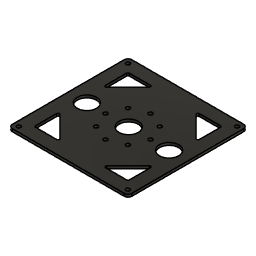
motor-holder (Autodesk Fusion 360 design; units mm, degrees)
Autodesk Fusion 360 part; units mm, degrees
sketch "Sketch1" plane through (0, 0, 0) normal (0, 0, 1) x (1, 0, 0)
  line L0 (-27, 30) -> (60, 30)
  line L1 (63, 27) -> (63, -60)
  line L2 (60, -63) -> (-27, -63)
  line L3 (-30, -60) -> (-30, 27)
  arc A0 (-27, 30) -> (-30, 27) centre (-27, 27) ccw
  arc A1 (63, 27) -> (60, 30) centre (60, 27) ccw
  arc A2 (-30, -60) -> (-27, -63) centre (-27, -60) ccw
  arc A3 (60, -63) -> (63, -60) centre (60, -60) ccw
  point P0 (-30, 30)
  point P1 (63, 30)
  point P2 (-30, -63)
  dimension "d1" = 93
  dimension "d2" = 93
  dimension "d3" = 3
  dimension "d4" = 3
  constraint horizontal L0
  constraint vertical L1
  constraint horizontal L2
  constraint vertical L3
  constraint coincident P0 L0
  constraint coincident P0 L3
  constraint tangent L0 A0
  constraint tangent L3 A0
  constraint coincident P1 L0
  constraint coincident P1 L1
  constraint tangent L0 A1
  constraint tangent L1 A1
  constraint coincident P2 L2
  constraint coincident P2 L3
  constraint tangent L2 A2
  constraint tangent L3 A2
  constraint equal A1 A2
  constraint tangent L1 A3
  constraint tangent L2 A3
  constraint equal A1 A3
  measures "d1" distance of P0 P1
  measures "d2" distance of P0 P2
  measures "d3" radius of A0
  measures "d4" radius of A1
extrude "Extrude1" add sketch "Sketch1" along normal blind 2
sketch "Sketch2" plane through (0, 0, 2) normal (0, 0, 1) x (-1, 0, 0)
  arc A0 (30, 60) -> (27, 63) centre (27, 60) ccw
  line L0 (27, 63) -> (-60, 63)
  arc A1 (-60, 63) -> (-63, 60) centre (-60, 60) ccw
  line L1 (-63, 60) -> (-63, -27)
  arc A2 (-63, -27) -> (-60, -30) centre (-60, -27) ccw
  line L2 (-60, -30) -> (27, -30)
  arc A3 (27, -30) -> (30, -27) centre (27, -27) ccw
  line L3 (30, -27) -> (30, 60)
  point P0 (26, -26)
  point P1 (-59, -26)
  point P2 (26, 59)
  point P3 (-60, 60)
  point P4 (-59, 59)
  point P5 (-57.2336, -24.9323)
  dimension "d18" = 85
  dimension "d19" = 4
  dimension "d20" = 4
  dimension "d21" = 4
  dimension "d22" = 4
  dimension "d23" = 4
  dimension "d24" = 4
  dimension "d25" = 85
  dimension "d26" = 4
  constraint coincident P3 A1.centre
  measures "d18" distance of P0 P1
  measures "d19" distance of L1 P1
  measures "d20" distance of L3 P0
  measures "d21" distance of L2 P0
  measures "d22" distance of L2 P1
  measures "d23" distance of L3 P2
  measures "d24" distance of L0 P2
  measures "d25" horizontal distance of P2 P4
  measures "d26" distance of L0 P4
hole "Hole2" at (59, -59, 2) at (-26, -59, 2) at (-26, 26, 2) at (59, 26, 2) direction (0, 0, -1) diameter 3 depth 2 tip angle 118
sketch "Sketch3" plane through (0, 0, 2) normal (0, 0, 1) x (-1, 0, 0)
  line L0 (-60, -30) -> (27, -30)
  line L1 (30, -27) -> (30, 60)
  line L2 (27, 63) -> (-60, 63)
  point P0 (-16.5, 16.5)
  point P1 (-16.5, -1)
  point P2 (1, 16.5)
  point P3 (-16.5, 34)
  point P4 (-34, 16.5)
  point P5 (-28.8744, 28.8744)
  point P6 (-4.1256, 28.8744)
  point P7 (-4.1256, 4.1256)
  point P8 (-28.8744, 4.1256)
  point P9 (-34, 16.5)
  point P10 (-16.5, 34)
  point P11 (1, 16.5)
  point P12 (-16.5, -1)
  point P13 (-28.8744, 4.1256)
  point P14 (-28.8744, 28.8744)
  point P15 (-4.1256, 28.8744)
  point P16 (-4.1256, 4.1256)
  point P17 (-16.5, -1)
  point P18 (-34, 16.5)
  point P19 (-16.5, 34)
  point P20 (1, 16.5)
  point P21 (-4.1256, 4.1256)
  point P22 (-28.8744, 4.1256)
  point P23 (-28.8744, 28.8744)
  point P24 (-4.1256, 28.8744)
  point P25 (1, 16.5)
  point P26 (-16.5, -1)
  point P27 (-34, 16.5)
  point P28 (-16.5, 34)
  point P29 (-4.1256, 28.8744)
  point P30 (-4.1256, 4.1256)
  point P31 (-28.8744, 4.1256)
  point P32 (-28.8744, 28.8744)
  dimension "d30" = 46.5
  dimension "d31" = 46.5
  dimension "d32" = 17.5
  dimension "d34" = 46.5
  dimension "d35" = 46.5
  dimension "d36" = 46.5
  dimension "d38" = 46.5
  dimension "d39" = 17.5
  dimension "d40" = 17.5
  dimension "d41" = 17.5
  dimension "d47" = 360
  measures "d30" distance of P0 L0
  measures "d31" distance of P0 L1
  measures "d32" horizontal distance of P0 P25
  measures "d34" distance of P26 L1
  measures "d35" distance of P27 L0
  measures "d36" distance of P25 L2
  measures "d38" distance of P28 L1
  measures "d39" distance of P0 P27
  measures "d40" distance of P0 P26
  measures "d41" distance of P0 P28
hole "Hole3" at (16.5, -34, 2) at (-1, -16.5, 2) at (16.5, 1, 2) at (34, -16.5, 2) at (16.5, -34, 2) at (4.1256, -28.8744, 2) at (4.1256, -4.1256, 2) at (28.8744, -28.8744, 2) at (28.8744, -4.1256, 2) direction (0, 0, -1) diameter 3 depth 25 tip angle 118
sketch "Sketch4" plane through (0, 0, 2) normal (0, 0, 1) x (-1, 0, 0)
sketch "Sketch5" plane through (0, 0, 2) normal (0, 0, 1) x (-1, 0, 0)
  circle A0 centre (-28.8744, 28.8744) radius 1.5
  circle A1 centre (-4.1256, 28.8744) radius 1.5
  circle A2 centre (-34, 16.5) radius 1.5
  circle A3 centre (1, 16.5) radius 1.5
  circle A4 centre (-16.5, 34) radius 1.5
  circle A5 centre (-16.5, -1) radius 1.5
  circle A6 centre (-4.1256, 4.1256) radius 1.5
  circle A7 centre (-28.8744, 4.1256) radius 1.5
  circle A8 centre (26, -26) radius 1.5
  circle A9 centre (-59, 59) radius 1.5
  circle A10 centre (26, 59) radius 1.5
  circle A11 centre (-59, -26) radius 1.5
  arc A12 (30, 60) -> (27, 63) centre (27, 60) ccw
  line L0 (27, 63) -> (-60, 63)
  arc A13 (-60, 63) -> (-63, 60) centre (-60, 60) ccw
  line L1 (-63, 60) -> (-63, -27)
  arc A14 (-63, -27) -> (-60, -30) centre (-60, -27) ccw
  line L2 (-60, -30) -> (27, -30)
  arc A15 (27, -30) -> (30, -27) centre (27, -27) ccw
  line L3 (30, -27) -> (30, 60)
  circle A16 centre (15.5, 16.5) radius 7.5
  circle A17 centre (-48.5, 16.5) radius 7.5
  dimension "d48" = 15
  dimension "d49" = 14.5
  dimension "d50" = 46.5
  dimension "d51" = 15
  dimension "d52" = 46.5
  dimension "d53" = 14.5
  measures "d48" diameter of A16
  measures "d49" distance of L3 A16.centre
  measures "d50" distance of L2 A16.centre
  measures "d51" diameter of A17
  measures "d52" distance of L2 A17.centre
  measures "d53" distance of L1 A17.centre
extrude "Extrude2" cut sketch "Sketch5" against normal blind 9 contours A16 | A17
sketch "Sketch6" plane through (0, 0, 2) normal (0, 0, 1) x (-1, 0, 0)
  circle A0 centre (-48.5, 16.5) radius 7.5
  circle A1 centre (15.5, 16.5) radius 7.5
  circle A2 centre (-28.8744, 28.8744) radius 1.5
  circle A3 centre (-4.1256, 28.8744) radius 1.5
  circle A4 centre (-34, 16.5) radius 1.5
  circle A5 centre (1, 16.5) radius 1.5
  circle A6 centre (-16.5, 34) radius 1.5
  circle A7 centre (-16.5, -1) radius 1.5
  circle A8 centre (-4.1256, 4.1256) radius 1.5
  circle A9 centre (-28.8744, 4.1256) radius 1.5
  circle A10 centre (26, -26) radius 1.5
  circle A11 centre (-59, 59) radius 1.5
  circle A12 centre (26, 59) radius 1.5
  circle A13 centre (-59, -26) radius 1.5
  arc A14 (30, 60) -> (27, 63) centre (27, 60) ccw
  line L0 (27, 63) -> (-60, 63)
  arc A15 (-60, 63) -> (-63, 60) centre (-60, 60) ccw
  line L1 (-63, 60) -> (-63, -27)
  arc A16 (-63, -27) -> (-60, -30) centre (-60, -27) ccw
  line L2 (-60, -30) -> (27, -30)
  arc A17 (27, -30) -> (30, -27) centre (27, -27) ccw
  line L3 (30, -27) -> (30, 60)
sketch "Sketch7" plane through (0, 0, 2) normal (0, 0, 1) x (-1, 0, 0)
  line L0 (19, -20) -> (2.4142, -20)
  line L1 (1.7071, -18.2929) -> (18.2929, -1.7071)
  line L2 (20, -19) -> (20, -2.4142)
  arc A0 (19, -20) -> (20, -19) centre (19, -19) ccw
  arc A1 (1.7071, -18.2929) -> (2.4142, -20) centre (2.4142, -19) ccw
  arc A2 (20, -2.4142) -> (18.2929, -1.7071) centre (19, -2.4142) ccw
  line L3 (-51.2929, 34.7071) -> (-34.7071, 51.2929)
  arc A3 (-34.7071, 51.2929) -> (-35.4142, 53) centre (-35.4142, 52) ccw
  line L4 (-52, 53) -> (-35.4142, 53)
  line L5 (-53, 52) -> (-53, 35.4142)
  arc A4 (-53, 35.4142) -> (-51.2929, 34.7071) centre (-52, 35.4142) ccw
  arc A5 (-52, 53) -> (-53, 52) centre (-52, 52) ccw
  line L6 (-60, -30) -> (27, -30)
  line L7 (-52, -20) -> (-35.4142, -20)
  arc A6 (-35.4142, -20) -> (-34.7071, -18.2929) centre (-35.4142, -19) ccw
  line L8 (-51.2929, -1.7071) -> (-34.7071, -18.2929)
  arc A7 (-51.2929, -1.7071) -> (-53, -2.4142) centre (-52, -2.4142) ccw
  line L9 (-53, -19) -> (-53, -2.4142)
  line L10 (1.7071, 51.2929) -> (18.2929, 34.7071)
  arc A8 (2.4142, 53) -> (1.7071, 51.2929) centre (2.4142, 52) ccw
  line L11 (19, 53) -> (2.4142, 53)
  arc A9 (20, 52) -> (19, 53) centre (19, 52) ccw
  line L12 (20, 52) -> (20, 35.4142)
  arc A10 (18.2929, 34.7071) -> (20, 35.4142) centre (19, 35.4142) ccw
  arc A11 (-53, -19) -> (-52, -20) centre (-52, -19) ccw
  point P0 (20, -20)
  point P1 (20, 0)
  point P2 (0, -20)
  point P3 (-52, -19)
  dimension "d56" = 1
  dimension "d61" = 1
  constraint horizontal L0
  constraint perpendicular L0 L2
  constraint tangent L0 A0
  constraint tangent L2 A0
  constraint tangent L0 A1
  constraint tangent L1 A1
  constraint equal A0 A1
  constraint tangent L1 A2
  constraint tangent L2 A2
  constraint equal A0 A2
  constraint tangent L7 A11
  constraint tangent L9 A11
  measures "d56" radius of A0
  measures "d61" radius of A11
extrude "Extrude3" cut sketch "Sketch7" against normal blind 5
sketch "Sketch8" plane through (0, 0, 0) normal (0, 0, 1) x (1, 0, 0)
  line L0 (60, 30) -> (-27, 30)
sketch "Sketch9" plane through (0, 0, 0) normal (0, 0, 1) x (1, 0, 0)
sketch "Sketch10" plane through (0, 0, 2) normal (0, 0, 1) x (-1, 0, 0)
  circle A0 centre (-17, 16.5) radius 7.5
  line L0 (-60, -30) -> (27, -30)
  dimension "d62" = 15
  dimension "d63" = 46.5
  measures "d62" diameter of A0
  measures "d63" distance of A0.centre L0
extrude "Extrude4" cut sketch "Sketch10" against normal blind 10
